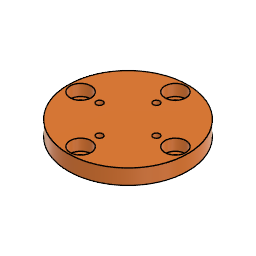
Franka and UR10 mount (Autodesk Fusion 360 design; units mm, degrees)
part number: 2026-03-03-19-08-19-558
Autodesk Fusion 360 part; units mm, degrees
sketch "Sketch1" plane through (0, 0, 0) normal (0, 0, 1) x (1, 0, 0)
  circle A0 centre (0, 0) radius 15 construction
  circle A1 centre (0, 15) radius 1.7
  circle A2 centre (-15, 0) radius 1.7
  circle A3 centre (0, -15) radius 1.7
  circle A4 centre (15, 0) radius 1.7
  circle A5 centre (0, 0) radius 25
  circle A6 centre (0, 25) radius 1.5 construction
  circle A7 centre (-25, 0) radius 1.5 construction
  circle A8 centre (0, -25) radius 1.5 construction
  circle A9 centre (25, 0) radius 1.5 construction
  circle A10 centre (0, 0) radius 31.5
  circle A11 centre (0, 0) radius 25 construction
  dimension "d426" = 30
  dimension "d427" = 3.4
  dimension "d429" = 360
  dimension "d430" = 50
  dimension "d432" = 3
  dimension "d442" = 63
  dimension "d443" = 50
  constraint coincident A0.centre A5.centre
  constraint coincident A0 A1.centre
  constraint concentric A0 A5
  constraint coincident A5 A6.centre
  constraint concentric A5 A10
  constraint concentric A5 A11
  measures "d426" diameter of A0
  measures "d427" diameter of A1
  measures "d430" diameter of A5
  measures "d432" diameter of A6
  measures "d442" diameter of A10
  measures "d443" diameter of A11
extrude "Extrude1" add sketch "Sketch1" along normal blind 8 contours A5 | A10
hole "Hole2" at (15, 0, 0) at (0, -15, 0) at (-15, 0, 0) at (0, 15, 0) direction (0, 0, 1) diameter 3.4 depth 9 tip angle 118 counterbore diameter 6.5 counterbore depth 3
sketch "Sketch2" plane through (0, 0, 8) normal (0, 0, 1) x (-1, 0, 0)
  circle A0 centre (-15, 0) radius 1.7
  circle A1 centre (15, 0) radius 1.7
  circle A2 centre (0, 15) radius 1.7
  circle A3 centre (0, -15) radius 1.7
  circle A4 centre (0, 0) radius 31.5
  circle A5 centre (0, 0) radius 25
  circle A6 centre (0, -25) radius 1.5 construction
  circle A7 centre (25, 0) radius 1.5 construction
  circle A8 centre (0, 25) radius 1.5 construction
  circle A9 centre (-25, 0) radius 1.5 construction
  dimension "d449" = 50
  dimension "d450" = 3
  dimension "d452" = 360
  constraint coincident A4.centre A5.centre
  constraint coincident A5 A6.centre
  measures "d449" diameter of A5
  measures "d450" diameter of A6
hole "Hole3" at (0, 25, 8) at (25, 0, 8) at (0, -25, 8) at (-25, 0, 8) direction (0, 0, -1) diameter 6.6 depth 9 tip angle 118 counterbore diameter 11 counterbore depth 6
equation "d426 = promjer_utori"
equation "d443 = promjer_silikona"
equation "promjer_prihvata = promjer_silikona - 10 mm"
equation "promjer_silikona = 50 mm"
equation "promjer_utori = promjer_prihvata - 10 mm"
named bodies: "Franka prihvat"
